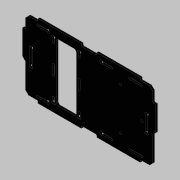
# Autodesk Inventor part: AK-C-C39-Main-Board
Saved by Autodesk Inventor 2016 (Build 200138000, 138)
## iProperties
Created: 2016-04-01
Part Number: AK-C-C39-Main-Board
Material: Generic
Document SubType Name: Modeling
Designer: admin
Density: 1 g/cm^3
Appearance: Smooth - Black
Author: admin
Autodesk Inventor part; units mm, degrees
ref_plane "YZ Plane" through (0, 0, 0) normal (1, 0, 0) x (0, 1, 0)
ref_plane "XZ Plane" through (0, 0, 0) normal (0, 1, 0) x (-1, 0, 0)
ref_plane "XY Plane" through (0, 0, 0) normal (0, 0, 1) x (1, 0, 0)
derived "SZOMK-AK-C-C39.ipt"
sketch "Sketch1" plane through (0, 0, 0) normal (0, 1, 0) x (-1, 0, 0)
  arc A0 (55.1118, 28.4761) -> (54.0511, 29.5368) centre (55.5, 29.925) ccw
  arc A1 (-54.0059, 29.7916) -> (-55.1118, 28.4761) centre (-55.5, 29.925) ccw
  arc A2 (54.0511, -29.5368) -> (55.1118, -28.4761) centre (55.5, -29.925) ccw
  arc A3 (-55.1118, -28.4761) -> (-54.0511, -29.5368) centre (-55.5, -29.925) ccw
  line L0 (55.5, 34.425) -> (-55.5, 34.425)
  line L1 (55.5, -34.425) -> (-55.5, -34.425)
  line L2 (33.1179, 0) -> (-42.957, 0) construction
  line L3 (0, -20.0068) -> (0, 12.0803) construction
  line L4 (-77.7331, -29.925) -> (-117.8042, -29.925) construction
  line L5 (-91.6184, 29.925) -> (-122.9166, 29.925) construction
  line L6 (55.5, -18.8016) -> (55.5, 12.0803) construction
  line L7 (-55.5, -18.8016) -> (-55.5, 16.5996) construction
  arc A4 (55.5, -34.425) -> (60, -29.925) centre (55.5, -29.925) ccw
  arc A5 (60, 29.925) -> (55.5, 34.425) centre (55.5, 29.925) ccw
  arc A6 (-55.5, 34.425) -> (-60, 29.925) centre (-55.5, 29.925) ccw
  arc A7 (-60, -29.925) -> (-55.5, -34.425) centre (-55.5, -29.925) ccw
  line L8 (57.5, 27.125) -> (57.5, 25.125)
  line L9 (57.5, 25.125) -> (55.5, 25.125)
  line L10 (55.5, 25.125) -> (55.5, 23.125)
  line L11 (55.5, 23.125) -> (57.5, 23.125)
  line L12 (57.5, 23.125) -> (57.5, 21.125)
  line L13 (57.5, 21.125) -> (55.5, 21.125)
  line L14 (55.5, 21.125) -> (55.5, 19.125)
  line L15 (55.5, 19.125) -> (57.8, 19.125)
  line L16 (57.8, 19.125) -> (57.8, -3.3607)
  line L17 (-57.5, 27.125) -> (-57.5, 25.125)
  line L18 (-57.5, 25.125) -> (-55.5, 25.125)
  line L19 (-55.5, 25.125) -> (-55.5, 23.125)
  line L20 (-55.5, 23.125) -> (-57.5, 23.125)
  line L21 (-57.5, 23.125) -> (-57.5, 21.125)
  line L22 (-57.5, 21.125) -> (-55.5, 21.125)
  line L23 (-55.5, 21.125) -> (-55.5, 19.125)
  line L24 (-55.5, 19.125) -> (-57.8, 19.125)
  line L25 (-57.8, 19.125) -> (-57.8, -3.3607)
  line L26 (57.5, 27.125) -> (54.9678, 27.125)
  line L27 (52.7, 29.3928) -> (52.7, 31.925)
  line L28 (52.7, 31.925) -> (50.7, 31.925)
  line L29 (50.7, 31.925) -> (50.7, 29.925)
  line L30 (50.7, 29.925) -> (48.7, 29.925)
  line L31 (48.7, 29.925) -> (48.7, 31.925)
  line L32 (48.7, 31.925) -> (46.7, 31.925)
  line L33 (46.7, 31.925) -> (46.7, 29.925)
  line L34 (46.7, 29.925) -> (44.7, 29.925)
  line L35 (44.7, 29.925) -> (44.7, 32.225)
  line L36 (44.7, 32.225) -> (5, 32.225)
  line L37 (5, 32.225) -> (5, 29.925)
  line L38 (5, 29.925) -> (3, 29.925)
  line L39 (3, 29.925) -> (3, 31.925)
  line L40 (3, 31.925) -> (1, 31.925)
  line L41 (1, 31.925) -> (1, 29.925)
  line L42 (1, 29.925) -> (-1, 29.925)
  line L43 (-1, 29.925) -> (-1, 31.925)
  line L44 (-1, 31.925) -> (-3, 31.925)
  line L45 (-3, 31.925) -> (-3, 29.925)
  line L46 (-3, 29.925) -> (-5, 29.925)
  line L47 (-5, 29.925) -> (-5, 32.225)
  line L48 (-5, 32.225) -> (-44.7, 32.225)
  line L49 (-44.7, 32.225) -> (-44.7, 29.925)
  line L50 (-44.7, 29.925) -> (-46.7, 29.925)
  line L51 (-46.7, 29.925) -> (-46.7, 32.225)
  line L52 (-46.7, 32.225) -> (-48.7, 32.225)
  line L53 (-48.7, 32.225) -> (-48.7, 29.925)
  line L54 (-48.7, 29.925) -> (-50.7, 29.925)
  line L55 (-50.7, 29.925) -> (-50.7, 32.225)
  line L56 (-50.7, 32.225) -> (-52.7, 32.225)
  line L57 (-52.7, 32.225) -> (-52.7, 29.6928)
  line L58 (-54.9678, 27.125) -> (-57.5, 27.125)
  line L59 (55.1118, 28.4761) -> (54.6142, 27.9786)
  line L60 (54.0511, 29.5368) -> (53.5536, 29.0392)
  line L61 (55.5, 29.925) -> (49.0175, 23.4425) construction
  arc A8 (52.7, 29.3928) -> (53.5536, 29.0392) centre (53.2, 29.3928) ccw
  arc A9 (54.6142, 27.9786) -> (54.9678, 27.125) centre (54.9678, 27.625) ccw
  line L62 (-55.1118, 28.4761) -> (-54.6142, 27.9786)
  line L63 (-54.0059, 29.7916) -> (-53.5536, 29.3392)
  arc A10 (-53.5536, 29.3392) -> (-52.7, 29.6928) centre (-53.2, 29.6928) ccw
  arc A11 (-54.9678, 27.125) -> (-54.6142, 27.9786) centre (-54.9678, 27.625) ccw
  line L64 (57.8, -3.3607) -> (55, -7.6074)
  line L65 (55, -7.6074) -> (55, -16.775)
  arc A12 (56.5, -18.525) -> (58.5, -18.525) centre (57.5, -19.275) ccw
  line L66 (58.5, -18.525) -> (58.5, -16.775)
  line L67 (56.5, -18.525) -> (56.5, -16.775)
  line L68 (55, -16.775) -> (56.5, -16.775)
  line L69 (58.5, -16.775) -> (60, -16.775)
  line L70 (57.5, -16.4962) -> (57.5, -11.7384) construction
  line L71 (-57.8, -3.3607) -> (-55, -7.6074)
  line L72 (-55, -7.6074) -> (-55, -16.775)
  arc A13 (-56.5, -15.025) -> (-58.5, -15.025) centre (-57.5, -14.275) ccw
  line L73 (-58.5, -15.025) -> (-58.5, -16.775)
  line L74 (-56.5, -15.025) -> (-56.5, -16.775)
  line L75 (-55, -16.775) -> (-56.5, -16.775)
  line L76 (-58.5, -16.775) -> (-60, -16.775)
  line L77 (-57.5, -20.9142) -> (-57.5, -16.6435) construction
  line L78 (44.7, -32.225) -> (5, -32.225)
  line L79 (5, -32.225) -> (5, -29.925)
  line L80 (5, -29.925) -> (3, -29.925)
  line L81 (3, -29.925) -> (3, -31.925)
  line L82 (3, -31.925) -> (1, -31.925)
  line L83 (1, -31.925) -> (1, -29.925)
  line L84 (1, -29.925) -> (-1, -29.925)
  line L85 (-1, -29.925) -> (-1, -31.925)
  line L86 (-1, -31.925) -> (-3, -31.925)
  line L87 (-3, -31.925) -> (-3, -29.925)
  line L88 (-3, -29.925) -> (-5, -29.925)
  line L89 (-5, -29.925) -> (-5, -32.225)
  line L90 (-5, -32.225) -> (-44.7, -32.225)
  line L91 (55, -17.425) -> (55, -25.125)
  line L92 (55, -25.125) -> (57.5, -25.125)
  line L93 (57.5, -25.125) -> (57.5, -27.125)
  line L94 (57.5, -27.125) -> (54.9678, -27.125)
  line L95 (52.7, -29.3928) -> (52.7, -31.925)
  line L96 (52.7, -31.925) -> (50.7, -31.925)
  line L97 (50.7, -31.925) -> (50.7, -29.925)
  line L98 (50.7, -29.925) -> (48.7, -29.925)
  line L99 (48.7, -29.925) -> (48.7, -31.925)
  line L100 (48.7, -31.925) -> (46.7, -31.925)
  line L101 (46.7, -31.925) -> (46.7, -29.925)
  line L102 (46.7, -29.925) -> (44.7, -29.925)
  line L103 (44.7, -29.925) -> (44.7, -32.225)
  line L104 (-44.7, -32.225) -> (-44.7, -29.925)
  line L105 (-44.7, -29.925) -> (-46.7, -29.925)
  line L106 (-46.7, -29.925) -> (-46.7, -31.925)
  line L107 (-46.7, -31.925) -> (-48.7, -31.925)
  line L108 (-48.7, -31.925) -> (-48.7, -29.925)
  line L109 (-48.7, -29.925) -> (-50.7, -29.925)
  line L110 (-50.7, -29.925) -> (-50.7, -31.925)
  line L111 (-50.7, -31.925) -> (-52.7, -31.925)
  line L112 (-52.7, -31.925) -> (-52.7, -29.3928)
  line L113 (-54.9678, -27.125) -> (-57.5, -27.125)
  line L114 (-57.5, -27.125) -> (-57.5, -25.125)
  line L115 (-57.5, -25.125) -> (-55, -25.125)
  line L116 (-55, -25.125) -> (-55, -17.425)
  line L117 (54.6142, -27.9786) -> (55.1118, -28.4761)
  line L118 (53.5536, -29.0392) -> (54.0511, -29.5368)
  arc A14 (54.9678, -27.125) -> (54.6142, -27.9786) centre (54.9678, -27.625) ccw
  arc A15 (53.5536, -29.0392) -> (52.7, -29.3928) centre (53.2, -29.3928) ccw
  line L119 (-54.0511, -29.5368) -> (-53.5536, -29.0392)
  line L120 (-55.1118, -28.4761) -> (-54.6142, -27.9786)
  arc A16 (-52.7, -29.3928) -> (-53.5536, -29.0392) centre (-53.2, -29.3928) ccw
  arc A17 (-54.6142, -27.9786) -> (-54.9678, -27.125) centre (-54.9678, -27.625) ccw
  line L121 (55, -17.425) -> (56.5, -17.425)
  line L122 (58.5, -17.425) -> (60, -17.425)
  line L123 (60, -29.925) -> (60, -17.425)
  line L124 (60, -16.775) -> (60, 29.925)
  line L125 (-55, -17.425) -> (-56.5, -17.425)
  line L126 (-56.5, -17.425) -> (-56.5, -16.775)
  line L127 (-58.5, -16.775) -> (-58.5, -17.425)
  line L128 (-58.5, -17.425) -> (-60, -17.425)
  line L129 (-60, -29.925) -> (-60, -17.425)
  line L130 (-60, -16.775) -> (-60, 29.925)
  point P0 (0, 0)
sketch "Sketch2" plane through (0, 0, 0) normal (0, 1, 0) x (-1, 0, 0)
  line L0 (51.25, -29) -> (44, -29)
  line L1 (43.25, -29.75) -> (43.25, -31)
  line L2 (43.25, -31) -> (6.5, -31)
  line L3 (6.5, -31) -> (6.5, -29.75)
  line L4 (5.75, -29) -> (-5.75, -29)
  line L5 (-6.5, -29.75) -> (-6.5, -31)
  line L6 (-6.5, -31) -> (-43.25, -31)
  line L7 (-43.25, -31) -> (-43.25, -29.75)
  line L8 (-44, -29) -> (-51.25, -29)
  line L9 (-51.25, -29) -> (-53.75, -26.5)
  line L10 (-53.75, -26.5) -> (-53.75, -5.5)
  line L11 (-53.75, -5.5) -> (-56.25, -3)
  line L12 (-56.25, -3) -> (-56.25, 18)
  line L13 (-56.25, 18) -> (-54.5, 18)
  line L14 (-53.75, 18.75) -> (-53.75, 26.5)
  line L15 (-53.75, 26.5) -> (-51.25, 29)
  line L16 (-51.25, 29) -> (-44, 29)
  line L17 (-43.25, 29.75) -> (-43.25, 31)
  line L18 (-43.25, 31) -> (-6.5, 31)
  line L19 (-6.5, 31) -> (-6.5, 29.75)
  line L20 (-5.75, 29) -> (5.75, 29)
  line L21 (6.5, 29.75) -> (6.5, 31)
  line L22 (43.25, 31) -> (43.25, 29.75)
  line L23 (43.25, 31) -> (6.5, 31)
  line L24 (44, 29) -> (51.25, 29)
  line L25 (51.25, 29) -> (53.75, 26.5)
  line L26 (53.75, 26.5) -> (53.75, 18.75)
  line L27 (54.5, 18) -> (56.25, 18)
  line L28 (56.25, 18) -> (56.25, -3)
  line L29 (56.25, -3) -> (53.75, -5.5)
  line L30 (53.75, -5.5) -> (53.75, -26.5)
  line L31 (53.75, -26.5) -> (51.25, -29)
  line L32 (44.7, -32.225) -> (5, -32.225) projected
  line L33 (5, -32.225) -> (5, -29.925) projected
  line L34 (5, -29.925) -> (3, -29.925) projected
  line L35 (44.7, -29.925) -> (44.7, -32.225) projected
  line L36 (46.7, -29.925) -> (44.7, -29.925) projected
  line L37 (52.7, -29.3928) -> (52.7, -31.925) projected
  arc A0 (53.5536, -29.0392) -> (52.7, -29.3928) centre (53.2, -29.3928) ccw projected
  arc A1 (54.9678, -27.125) -> (54.6142, -27.9786) centre (54.9678, -27.625) ccw projected
  line L38 (55, -17.425) -> (55, -25.125) projected
  line L39 (0, -20.0068) -> (0, 12.0803) construction
  line L40 (33.1179, 0) -> (-42.957, 0) construction
  line L41 (57.8, 19.125) -> (57.8, -3.3607) projected
  line L42 (57.8, -3.3607) -> (55, -7.6074) projected
  line L43 (55.5, 19.125) -> (57.8, 19.125) projected
  line L44 (55.5, 29.925) -> (49.0175, 23.4425) construction
  line L45 (25.75, -24.5) -> (12.75, -24.5)
  line L46 (12.75, 24.5) -> (25.75, 24.5)
  line L47 (3.3524, -20) -> (-16.6476, -20) construction
  line L48 (-16.6476, -20) -> (-16.6476, 20) construction
  line L49 (-16.6476, 20) -> (3.3524, 20) construction
  line L50 (3.3524, 20) -> (3.3524, -20) construction
  line L51 (-23.9878, -15) -> (-31.9878, -15) construction
  line L52 (-31.9878, -15) -> (-31.9878, -7) construction
  line L53 (-31.9878, -7) -> (-23.9878, -7) construction
  line L54 (-23.9878, -7) -> (-23.9878, -15) construction
  line L55 (-34.9878, -15) -> (-42.9878, -15) construction
  line L56 (-42.9878, -15) -> (-42.9878, -7) construction
  line L57 (-42.9878, -7) -> (-34.9878, -7) construction
  line L58 (-34.9878, -7) -> (-34.9878, -15) construction
  line L59 (-23.9878, -4) -> (-31.9878, -4) construction
  line L60 (-31.9878, -4) -> (-31.9878, 4) construction
  line L61 (-31.9878, 4) -> (-23.9878, 4) construction
  line L62 (-23.9878, 4) -> (-23.9878, -4) construction
  line L63 (-34.9878, -4) -> (-42.9878, -4) construction
  line L64 (-42.9878, -4) -> (-42.9878, 4) construction
  line L65 (-42.9878, 4) -> (-34.9878, 4) construction
  line L66 (-34.9878, 4) -> (-34.9878, -4) construction
  line L67 (-23.9878, 7) -> (-31.9878, 7) construction
  line L68 (-31.9878, 7) -> (-31.9878, 15) construction
  line L69 (-31.9878, 15) -> (-23.9878, 15) construction
  line L70 (-23.9878, 15) -> (-23.9878, 7) construction
  line L71 (-34.9878, 7) -> (-42.9878, 7) construction
  line L72 (-42.9878, 7) -> (-42.9878, 15) construction
  line L73 (-42.9878, 15) -> (-34.9878, 15) construction
  line L74 (-34.9878, 15) -> (-34.9878, 7) construction
  line L75 (25.75, -22.5) -> (12.75, -22.5) construction
  line L76 (12.75, -22.5) -> (12.75, -9.5) construction
  line L77 (12.75, -9.5) -> (25.75, -9.5) construction
  line L78 (25.75, -9.5) -> (25.75, -22.5) construction
  line L79 (25.75, -6.5) -> (12.75, -6.5) construction
  line L80 (12.75, -6.5) -> (12.75, 6.5) construction
  line L81 (12.75, 6.5) -> (25.75, 6.5) construction
  line L82 (25.75, 6.5) -> (25.75, -6.5) construction
  line L83 (25.75, 9.5) -> (12.75, 9.5) construction
  line L84 (12.75, 9.5) -> (12.75, 22.5) construction
  line L85 (12.75, 22.5) -> (25.75, 22.5) construction
  line L86 (25.75, 22.5) -> (25.75, 9.5) construction
  line L87 (31.9633, -16) -> (17.7262, -16) construction
  line L88 (31.9633, 16) -> (18.8213, 16) construction
  line L89 (19.25, -23.7063) -> (19.25, 24.6931) construction
  arc A2 (10.75, -22.5) -> (12.75, -24.5) centre (12.75, -22.5) ccw
  arc A3 (25.75, -24.5) -> (27.75, -22.5) centre (25.75, -22.5) ccw
  arc A4 (12.75, 24.5) -> (10.75, 22.5) centre (12.75, 22.5) ccw
  arc A5 (27.75, 22.5) -> (25.75, 24.5) centre (25.75, 22.5) ccw
  line L90 (55, -25.125) -> (-54.9956, -25.125) construction
  line L91 (55.5, 25.125) -> (55.5, 23.125) projected
  line L92 (57.5, 25.125) -> (55.5, 25.125) projected
  line L93 (-57.5, 25.125) -> (-55.5, 25.125) projected
  line L94 (-55.5, 25.125) -> (-55.5, 23.125) projected
  line L95 (-57.5, -25.125) -> (-55, -25.125) projected
  line L96 (-55, -25.125) -> (-55, -17.425) projected
  line L97 (55, -25.125) -> (57.5, -25.125) projected
  line L98 (55.5, 25.125) -> (-55.5, 25.125) construction
  line L99 (48.25, -6.5) -> (48.25, 6.5)
  line L100 (50, -6.5) -> (50, 6.5)
  line L101 (50, -8) -> (48.25, -8)
  line L102 (50, 8) -> (48.25, 8)
  arc A6 (50, -8) -> (50, -6.5) centre (50, -7.25) ccw
  arc A7 (48.25, -6.5) -> (48.25, -8) centre (48.25, -7.25) ccw
  arc A8 (50, 6.5) -> (50, 8) centre (50, 7.25) ccw
  arc A9 (48.25, 8) -> (48.25, 6.5) centre (48.25, 7.25) ccw
  line L103 (-47.75, -6.5) -> (-47.75, 6.5)
  line L104 (-49.5, 8) -> (-47.75, 8)
  line L105 (-49.5, 6.5) -> (-49.5, -6.5)
  line L106 (-49.5, -8) -> (-47.75, -8)
  arc A10 (-47.75, -8) -> (-47.75, -6.5) centre (-47.75, -7.25) ccw
  arc A11 (-49.5, -6.5) -> (-49.5, -8) centre (-49.5, -7.25) ccw
  arc A12 (-47.75, 6.5) -> (-47.75, 8) centre (-47.75, 7.25) ccw
  arc A13 (-49.5, 8) -> (-49.5, 6.5) centre (-49.5, 7.25) ccw
  line L107 (43.75, -27) -> (35.5, -27)
  line L108 (33.75, -27) -> (33.75, -25.25)
  line L109 (35.5, -25.25) -> (43.75, -25.25)
  line L110 (-11, -27) -> (-19.25, -27)
  line L111 (-19.25, -25.25) -> (-11, -25.25)
  line L112 (-9.25, -25.25) -> (-9.25, -27)
  line L113 (-34.25, -27) -> (-44.25, -27)
  line L114 (-44.25, -25.25) -> (-34.25, -25.25)
  line L115 (-44.25, 25.25) -> (-34.25, 25.25)
  line L116 (-34.25, 27) -> (-44.25, 27)
  line L117 (-10.75, 25.25) -> (-19.25, 25.25)
  line L118 (-19.25, 27) -> (-10.75, 27)
  line L119 (-9.25, 27) -> (-9.25, 25.25)
  line L120 (43.75, 25.25) -> (35.25, 25.25)
  line L121 (33.75, 25.25) -> (33.75, 27)
  line L122 (35.25, 27) -> (43.75, 27)
  arc A14 (33.75, -27) -> (35.5, -27) centre (34.625, -27) ccw
  arc A15 (35.5, -25.25) -> (33.75, -25.25) centre (34.625, -25.25) ccw
  arc A16 (-11, -27) -> (-9.25, -27) centre (-10.125, -27) ccw
  arc A17 (-9.25, -25.25) -> (-11, -25.25) centre (-10.125, -25.25) ccw
  arc A18 (33.75, 25.25) -> (35.25, 25.25) centre (34.5, 25.25) ccw
  arc A19 (35.25, 27) -> (33.75, 27) centre (34.5, 27) ccw
  arc A20 (-9.25, 27) -> (-10.75, 27) centre (-10, 27) ccw
  arc A21 (-10.75, 25.25) -> (-9.25, 25.25) centre (-10, 25.25) ccw
  line L123 (27.75, 22.5) -> (27.75, -22.5)
  line L124 (-34.9878, 7) -> (-42.9878, 15) construction
  line L125 (-31.9878, 7) -> (-23.9878, 15) construction
  line L126 (-31.9878, -7) -> (-23.9878, -15) construction
  line L127 (-34.9878, -7) -> (-42.9878, -15) construction
  line L128 (10.75, 7.999) -> (10.75, 8)
  line L129 (10.75, -22.5) -> (10.75, 22.5)
  arc A22 (43.75, 25.25) -> (43.75, 27) centre (43.75, 26.125) ccw
  arc A23 (-19.25, 27) -> (-19.25, 25.25) centre (-19.25, 26.125) ccw
  arc A24 (-34.25, 25.25) -> (-34.25, 27) centre (-34.25, 26.125) ccw
  arc A25 (-44.25, 27) -> (-44.25, 25.25) centre (-44.25, 26.125) ccw
  arc A26 (43.75, -27) -> (43.75, -25.25) centre (43.75, -26.125) ccw
  arc A27 (-19.25, -25.25) -> (-19.25, -27) centre (-19.25, -26.125) ccw
  arc A28 (-34.25, -27) -> (-34.25, -25.25) centre (-34.25, -26.125) ccw
  arc A29 (-44.25, -25.25) -> (-44.25, -27) centre (-44.25, -26.125) ccw
  line L130 (31, 25) -> (29.25, 25)
  line L131 (31, 23.5) -> (31, 20)
  line L132 (29.25, 20) -> (29.25, 23.5)
  arc A30 (31, 23.5) -> (31, 25) centre (31, 24.25) ccw
  arc A31 (29.25, 25) -> (29.25, 23.5) centre (29.25, 24.25) ccw
  arc A32 (29.25, 20) -> (31, 20) centre (30.125, 20) ccw
  line L133 (29.25, -20) -> (29.25, -23.25)
  line L134 (29.25, -25) -> (31, -25)
  line L135 (31, -23.25) -> (31, -20)
  arc A33 (31, -25) -> (31, -23.25) centre (31, -24.125) ccw
  arc A34 (29.25, -23.25) -> (29.25, -25) centre (29.25, -24.125) ccw
  arc A35 (31, -20) -> (29.25, -20) centre (30.125, -20) ccw
  line L136 (9.25, 25) -> (7.5, 25)
  line L137 (7.5, 23.5) -> (7.5, 20)
  line L138 (9.25, 20) -> (9.25, 23.5)
  line L139 (7.5, -20) -> (7.5, -23.25)
  line L140 (7.5, -25) -> (9.25, -25)
  line L141 (9.25, -23.25) -> (9.25, -20)
  arc A36 (9.25, -20) -> (7.5, -20) centre (8.375, -20) ccw
  arc A37 (9.25, -25) -> (9.25, -23.25) centre (9.25, -24.125) ccw
  arc A38 (7.5, -23.25) -> (7.5, -25) centre (7.5, -24.125) ccw
  arc A39 (7.5, 20) -> (9.25, 20) centre (8.375, 20) ccw
  arc A40 (9.25, 23.5) -> (9.25, 25) centre (9.25, 24.25) ccw
  arc A41 (7.5, 25) -> (7.5, 23.5) centre (7.5, 24.25) ccw
  line L142 (29.25, 4) -> (29.25, -4)
  line L143 (31, -4) -> (31, 4)
  line L144 (7.5, 4) -> (7.5, -4)
  line L145 (9.25, -4) -> (9.25, 4)
  arc A42 (31, 4) -> (29.25, 4) centre (30.125, 4) ccw
  arc A43 (29.25, -4) -> (31, -4) centre (30.125, -4) ccw
  arc A44 (9.25, 4) -> (7.5, 4) centre (8.375, 4) ccw
  arc A45 (7.5, -4) -> (9.25, -4) centre (8.375, -4) ccw
  line L146 (-22.75, 30.3253) -> (-30.75, 30.3253) construction
  line L147 (-30.75, 30.3253) -> (-30.75, 22.4164) construction
  line L148 (-30.75, 22.4164) -> (-22.75, 22.4164) construction
  line L149 (-22.75, 22.4164) -> (-22.75, 30.3253) construction
  line L150 (-26.75, 29.9722) -> (-26.75, 20.9797) construction
  arc A46 (6.5, -29.75) -> (5.75, -29) centre (5.75, -29.75) ccw
  arc A47 (-5.75, -29) -> (-6.5, -29.75) centre (-5.75, -29.75) ccw
  arc A48 (-43.25, -29.75) -> (-44, -29) centre (-44, -29.75) ccw
  arc A49 (-54.5, 18) -> (-53.75, 18.75) centre (-54.5, 18.75) ccw
  arc A50 (-44, 29) -> (-43.25, 29.75) centre (-44, 29.75) ccw
  arc A51 (-6.5, 29.75) -> (-5.75, 29) centre (-5.75, 29.75) ccw
  arc A52 (5.75, 29) -> (6.5, 29.75) centre (5.75, 29.75) ccw
  arc A53 (43.25, 29.75) -> (44, 29) centre (44, 29.75) ccw
  arc A54 (53.75, 18.75) -> (54.5, 18) centre (54.5, 18.75) ccw
  arc A55 (44, -29) -> (43.25, -29.75) centre (44, -29.75) ccw
  line L151 (57.5, 27.125) -> (57.5, 25.125) projected
  line L152 (-57.5, 27.125) -> (-57.5, 25.125) projected
  point P0 (25.75, -16)
  point P1 (25.75, 16)
  point P2 (19.25, -22.5)
  point P3 (19.25, -24.5)
  point P4 (27.75, 0)
  point P5 (10.75, 0)
  point P6 (-26.75, 30.3253)
  point P7 (-26.75, 18)
  point P8 (-26.75, -18)
  point P9 (-44.75, 0)
  dimension "d10" = 13
  dimension "d14" = 8
  dimension "d15" = 2
  dimension "d16" = 49
  dimension "d26" = 1.5
  dimension "d28" = 1.75
  dimension "d43" = 20
  dimension "d44" = 40
  dimension "d46" = 3
  dimension "d50" = 29
  dimension "d52" = 6.25
  dimension "d53" = 17
  dimension "d54" = 10
  dimension "d55" = 10
  dimension "d56" = 5
  dimension "d57" = 10
  dimension "d58" = 10
  dimension "d59" = 15
  dimension "d60" = 1.75
  dimension "d61" = 67
  dimension "d63" = 43
  dimension "d68" = 16
  dimension "d69" = 8
  dimension "d70" = 8
  dimension "d73" = 10
  dimension "d74" = 2.5
  dimension "d75" = 107.5
  dimension "d78" = 1.75
  dimension "d79" = 20
  dimension "d80" = 0.25
  dimension "d81" = 62
  dimension "d83" = 29
  dimension "d84" = 18
  dimension "d85" = 13
  dimension "d86" = 13
  dimension "d87" = 21
  dimension "d88" = 3
  dimension "d89" = 3
  dimension "d90" = 18
  dimension "d91" = 3
  dimension "d99" = 8
  dimension "d101" = 13.75
  dimension "d102" = 13.25
  dimension "d103" = 2.75
  dimension "d104" = 4.5
  dimension "d105" = 20
  dimension "d106" = 16
  constraints: 262 end point, 108 point on circle, 83 tangent, 63 point on line, 54 centre point, 39 parallel, 37 equal radius, 37 perpendicular, 25 horizontal, 18 collinear, 15 equal length, 7 midpoint, 6 horizontal alignment, 5 vertical, 5 vertical alignment, 4 symmetric about line, 22 other
  measures "d10" distance of L75.end L76.end
  measures "d14" distance of L51.start L51.end
  measures "d15" radius of A2
  measures "d16" distance between parallel lines of L46 L45
  measures "d26" diameter of A6
  measures "d28" distance of L101.start L101.end
  measures "d43" distance of L48.end L49.end
  measures "d44" distance of L47.end L48.end
  measures "d46" distance between parallel lines of L74 L68
  measures "d50" distance between parallel lines of L89 L99
  measures "d52" distance between parallel lines of L100 L28
  measures "d53" distance between parallel lines of L129 L123
  measures "d54" distance between parallel lines of L132 L89
  measures "d55" distance from line of L121 A22.centre
  measures "d56" distance from line of A32.centre L130
  measures "d57" distance from line of L119 A23.centre
  measures "d58" distance of A25.centre A24.centre
  measures "d59" distance of A24.centre A23.centre
  measures "d60" distance between parallel lines of L105 L103
  measures "d61" distance between parallel lines of L103 L89
  measures "d63" distance between parallel lines of L119 L121
  measures "d68" distance between parallel lines of L40 L88
  measures "d69" distance of A43.centre A42.centre
  measures "d70" distance between parallel lines of L147 L149
  measures "d73" distance from line of A22.centre L26
  measures "d74" distance between parallel lines of L28 L26
  measures "d75" distance between parallel lines of L14 L26
  measures "d78" distance between parallel lines of L122 L120
  measures "d79" distance from line of A32.centre L40
  measures "d80" distance between parallel lines of L109 L134
  measures "d81" distance between parallel lines of L2 L23
  measures "d83" distance between parallel lines of L0 L40
  measures "d84" distance between parallel lines of L40 L13
  measures "d85" distance between parallel lines of L22 L28
  measures "d86" distance between parallel lines of L19 L21
  measures "d87" distance of L29.end L30.end
  measures "d88" distance between parallel lines of L67 L61
  measures "d89" distance between parallel lines of L59 L53
  measures "d90" distance from line of L40 point (-26.75, 18)
  measures "d91" distance from line of point (-44.75, 0) L103
  measures "d99" distance from line of L22 L24.end
  measures "d101" distance from line of L151 A22.centre
  measures "d102" distance from line of L152 A25.centre
  measures "d103" distance between parallel lines of L121 L131
  measures "d104" distance from line of A22.centre L99
  measures "d105" distance between parallel lines of L138 L132
  measures "d106" distance between parallel lines of L101 L102
extrude "Extrusion1" add sketch "Sketch2" along normal blind 1.6
hole "Hole1" at (26.75, 0, 18) at (26.75, 0, -18) at (44.75, 0, 0) direction (0, 1, 0) diameter 2 end through all
equation "\"d22\" = d20"
equation "\"d24\" = d20"
equation "\"d20\" = 1.6"
body "Solid1"
